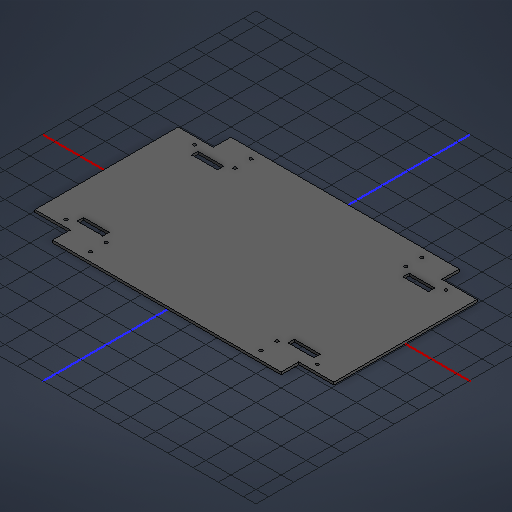
# Autodesk Inventor part: 000.001.002 - Днище
Saved by Autodesk Inventor 2025 (Build 290162000, 162)
## iProperties
Created: 2022-02-23
Part Number: 000.001.002 - Днище
Material: Типовые
Document SubType Name: Modeling
Designer: Petrov Ivan
Density: 1 g/cm^3
Appearance: По умолчанию(1)
Author: Petrov Ivan
Autodesk Inventor part; units mm, degrees
ref_plane "YZ Plane" through (0, 0, 0) normal (1, 0, 0) x (0, 1, 0)
ref_plane "XZ Plane" through (0, 0, 0) normal (0, 1, 0) x (-1, 0, 0)
ref_plane "XY Plane" through (0, 0, 0) normal (0, 0, 1) x (1, 0, 0)
sketch "Эскиз1" plane through (0, 0, 0) normal (0, 1, 0) x (-1, 0, 0)
  line L0 (-238, 142) -> (238, 142)
  line L1 (238, 142) -> (238, -142)
  line L2 (238, -142) -> (-238, -142)
  line L3 (-238, -142) -> (-238, 142)
  line L4 (-238, 142) -> (238, -142) construction
  line L5 (238, 142) -> (-238, -142) construction
  circle A0 centre (-139.231, 22.646) radius 2
  point P0 (0, 0)
  dimension "d0" = 476
  dimension "d1" = 284
  dimension "d10" = 4
  constraints: 12 end point, 2 midpoint, 2 parallel, 1 centre point, 1 horizontal, 1 perpendicular
  measures "d0" distance of L1.end L2.end
  measures "d1" distance of L0.end L1.end
  measures "d10" diameter of A0
extrude "Выдавливание1" add sketch "Эскиз1" along normal blind 4 contours L0 L1 L2 L3 | A0
sketch "Эскиз2" plane through (0, 4, 0) normal (0, 1, 0) x (1, 0, 0)
  line L0 (-238, -142) -> (238, -142) projected
  line L1 (-238, -142) -> (-182, -142)
  line L2 (-182, -142) -> (-182, -114)
  line L3 (-182, -114) -> (-238, -114)
  line L4 (-238, -114) -> (-238, -142)
  point P0 (0, 0)
  dimension "d4" = 56
  dimension "d5" = 28
  constraints: 8 end point, 2 parallel, 1 horizontal, 1 perpendicular
  measures "d4" distance of L3.end L2.end
  measures "d5" distance of L2.end L1.end
extrude "Выдавливание2" cut sketch "Эскиз2" against normal blind 4
mirror "Зеркальное отражение1" about plane through (0, 0, 0) normal (1, 0, 0) of "Выдавливание2"
mirror "Зеркальное отражение2" about plane through (0, 0, 0) normal (0, 0, 1) of "Выдавливание2", "Зеркальное отражение1"
sketch "Эскиз9" plane through (0, 0, 0) normal (0, -1, 0) x (1, 0, 0)
  circle A0 centre (-200, -128) radius 2.35 projected
  circle A1 centre (-136, -128) radius 2.35 projected
  circle A2 centre (-136, -128) radius 2.35 projected
  circle A3 centre (-136, -128) radius 2.35 projected
  circle A4 centre (-136, -102.6) radius 2.35 projected
  circle A5 centre (-200, -102.6) radius 2.35 projected
  circle A6 centre (-136, 102.6) radius 2.35 projected
  circle A7 centre (-136, 128) radius 2.35 projected
  circle A8 centre (-200, 102.6) radius 2.35 projected
  circle A9 centre (-200, 102.6) radius 2.35 projected
  circle A10 centre (-200, 102.6) radius 2.35 projected
  circle A11 centre (-200, 128) radius 2.35 projected
  circle A12 centre (200, 102.6) radius 2.35 projected
  circle A13 centre (200, 128) radius 2.35 projected
  circle A14 centre (136, 128) radius 2.35 projected
  circle A15 centre (136, 102.6) radius 2.35 projected
  circle A16 centre (200, -102.6) radius 2.35 projected
  circle A17 centre (200, -128) radius 2.35 projected
  circle A18 centre (136, -102.6) radius 2.35 projected
  circle A19 centre (136, -128) radius 2.35 projected
  point P0 (0, 0)
extrude "Выдавливание9" cut sketch "Эскиз9" against normal blind 10
sketch "Эскиз10" plane through (0, 0, 0) normal (0, -1, 0) x (1, 0, 0)
  line L0 (188.5, -86.25) -> (147.5, -86.25) projected
  line L1 (188.5, -96.25) -> (188.5, -86.25) projected
  line L2 (147.5, -96.25) -> (147.5, -86.25) projected
  line L3 (147.5, 96.25) -> (147.5, 86.25) projected
  line L4 (147.5, 86.25) -> (188.5, 86.25) projected
  line L5 (188.5, 96.25) -> (188.5, 86.25) projected
  line L6 (-188.5, 96.25) -> (-188.5, 86.25) projected
  line L7 (-188.5, 86.25) -> (-147.5, 86.25) projected
  line L8 (-147.5, 96.25) -> (-147.5, 86.25) projected
  line L9 (-188.5, -96.25) -> (-188.5, -86.25) projected
  line L10 (-147.5, -86.25) -> (-188.5, -86.25) projected
  line L11 (-147.5, -96.25) -> (-147.5, -86.25) projected
  line L12 (-188.5, 96.25) -> (-147.5, 96.25)
  line L13 (-147.5, 96.25) -> (-147.5, 86.25)
  line L14 (-147.5, 86.25) -> (-188.5, 86.25)
  line L15 (-188.5, 86.25) -> (-188.5, 96.25)
  line L16 (147.5, 96.25) -> (188.5, 96.25)
  line L17 (188.5, 96.25) -> (188.5, 86.25)
  line L18 (188.5, 86.25) -> (147.5, 86.25)
  line L19 (147.5, 86.25) -> (147.5, 96.25)
  line L20 (147.5, -96.25) -> (188.5, -96.25)
  line L21 (188.5, -96.25) -> (188.5, -86.25)
  line L22 (188.5, -86.25) -> (147.5, -86.25)
  line L23 (147.5, -86.25) -> (147.5, -96.25)
  line L24 (-188.5, -96.25) -> (-147.5, -96.25)
  line L25 (-147.5, -96.25) -> (-147.5, -86.25)
  line L26 (-147.5, -86.25) -> (-188.5, -86.25)
  line L27 (-188.5, -86.25) -> (-188.5, -96.25)
  point P0 (0, 0)
  constraints: 32 end point, 8 parallel, 4 horizontal, 4 perpendicular
extrude "Выдавливание10" cut sketch "Эскиз10" against normal blind 10
